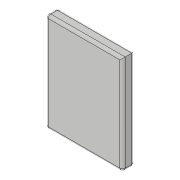
# Autodesk Inventor part: 328 Adafruit 2.5 Ah Lithium Battery
Saved by Autodesk Inventor 2018.3 (Build 223284000, 284)
## iProperties
Created: 2018-12-11
Part Number: 328 Adafruit 2.5 Ah Lithium Battery
Material: Generic
Document SubType Name: Modeling
Designer: tei06398
Mass: 19.4422 g
Surface Area: 67.3583 cm^2
Volume: 19.4422 cm^3
Density: 1 g/cm^3
Appearance: Default
Author: tei06398
Autodesk Inventor part; units mm, degrees
ref_plane "YZ Plane" through (0, 0, 0) normal (1, 0, 0) x (0, 1, 0)
ref_plane "XZ Plane" through (0, 0, 0) normal (0, 1, 0) x (-1, 0, 0)
ref_plane "XY Plane" through (0, 0, 0) normal (0, 0, 1) x (1, 0, 0)
sketch "Sketch1" plane through (0, 0, 0) normal (0, 0, 1) x (1, 0, 0)
  line L0 (0, 0) -> (46.355, 0)
  line L1 (46.355, 0) -> (46.355, 59.69)
  line L2 (46.355, 59.69) -> (0, 59.69)
  line L3 (0, 59.69) -> (0, 0)
  dimension "d0" = 46.355
  dimension "d1" = 59.69
  constraints: 8 end point, 2 parallel, 1 horizontal, 1 perpendicular
  measures "d0" distance of L2.end L1.end
  measures "d1" distance of L1.end L0.end
extrude "Extrusion1" add sketch "Sketch1" against normal blind 7.112
fillet "Fillet1" radius 1.5875 11 edges at (0, 29.845, 0) (23.1775, 59.69, 0) (46.355, 29.845, 0) (23.1775, 0, 0) (23.1775, 59.69, -7.112) (46.355, 29.845, -7.112) (0, 29.845, -7.112) (23.1775, 0, -7.112) (46.355, 0, -3.556) (0, 59.69, -3.556) (0, 0, -3.556)
body "Solid1"
